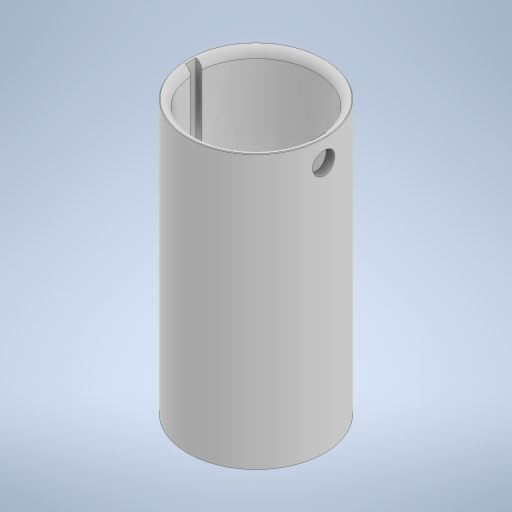
# Autodesk Inventor part: V1.0-battery-holder-A
Saved by Autodesk Inventor 2023 (Build 270158030, 158C)
## iProperties
Created: 2023-04-27
Part Number: V1.0-battery-holder-A
Material: Generic
Document SubType Name: Modeling
Designer: Imogen Heard
Density: 1 g/cm^3
Appearance: Default
Author: Imogen Heard
Autodesk Inventor part; units mm, degrees
ref_plane "YZ Plane" through (0, 0, 0) normal (1, 0, 0) x (0, 1, 0)
ref_plane "XZ Plane" through (0, 0, 0) normal (0, 1, 0) x (-1, 0, 0)
sketch "Sketch1" plane through (0, 0, 0) normal (0, 1, 0) x (-1, 0, 0)
  circle A0 centre (0, 0) radius 12.5
  dimension "d0" = 25
  constraints: 1 centre point, 1 coincident
  measures "d0" diameter of A0
extrude "Extrusion1" add sketch "Sketch1" along normal blind 50
sketch "Sketch2" plane through (0, 50, 0) normal (0, 1, 0) x (1, 0, 0)
  circle A0 centre (0, 0) radius 11
  circle A1 centre (0, 0) radius 12.5 projected
  line L0 (-12, -1) -> (-10.9545, -1)
  line L1 (-10.9545, 1) -> (-12, 1)
  line L2 (-12, 1) -> (-12, -1)
  point P0 (-12, 0)
  dimension "d3" = 22
  dimension "d4" = 12
  dimension "d5" = 1
  dimension "d6" = 1
  dimension "d7" = 1.0455
  constraints: 6 end point, 2 point on circle, 1 centre point, 1 concentric, 1 horizontal, 1 midpoint, 1 parallel
  measures "d3" diameter of A0
  measures "d4" distance from line of point (0, 0) L2
  measures "d5" distance from line of point (0, 0) L0
  measures "d6" distance from line of point (0, 0) L1
  measures "d7" horizontal distance of L1.start point (-12, 0)
extrude "Extrusion2" cut sketch "Sketch2" against normal blind 47 contours A0 | A0 L0 L2 L1
sketch "Sketch3" plane through (0, 3, 0) normal (0, 1, 0) x (1, 0, 0)
  circle A0 centre (0, 0) radius 10
  arc A1 (-10.9545, -1) -> (-10.9545, 1) centre (0, 0) ccw projected
  dimension "d10" = 20
  constraints: 1 centre point, 1 concentric
  measures "d10" diameter of A0
extrude "Extrusion3" add sketch "Sketch3" along normal blind 41 separate body
ref_plane "Work Plane1" through (12.5, 0, 0) normal (1, 0, 0) x (0, 0, -1)
sketch "Sketch4" plane through (12.5, 0, 0) normal (1, 0, 0) x (0, 0, -1)
  circle A0 centre (0, 46) radius 2
  line L0 (-11, 50) -> (11, 50) projected
  point P0 (0, 0)
  point P1 (0, 50)
  point P2 (1, 50)
  point P3 (-1, 50)
  dimension "d13" = 4
  dimension "d14" = 4
  constraints: 1 centre point, 1 midpoint, 1 vertical alignment
  measures "d13" diameter of A0
  measures "d14" distance from line of L0 A0.centre
extrude "Extrusion4" cut sketch "Sketch4" against normal blind 3
sketch "Sketch5" plane through (0, 50, 0) normal (0, 1, 0) x (1, 0, 0)
  line L0 (11.5, -1.3) -> (10.9229, -1.3)
  line L1 (10.9229, 1.3) -> (11.5, 1.3)
  line L2 (11.5, 1.3) -> (11.5, -1.3)
  arc A0 (-10.9545, -1) -> (-10.9545, 1) centre (0, 0) ccw projected
  point P0 (11, 0)
  dimension "d17" = 1.3
  dimension "d18" = 1.3
  dimension "d19" = 0.5
  constraints: 6 end point, 3 point on circle, 1 horizontal, 1 parallel
  measures "d17" distance from line of point (0, 0) L0
  measures "d18" distance from line of L1 point (0, 0)
  measures "d19" distance from line of L2 point (11, 0)
extrude "Extrusion5" cut sketch "Sketch5" against normal blind 3
fillet "Fillet1" radius 1.5 2 edges at (-0.1508, 50, -10.999) (-0.1508, 50, 10.999)
fillet "Fillet2" radius 0.1 2 edges at (-1.3904, 50, 12.4224) (1.3904, 50, -12.4224)
